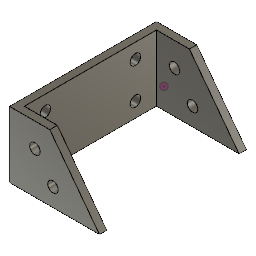
updated_housing_clamp_for_motor v3 (Autodesk Fusion 360 design; units mm, degrees)
Autodesk Fusion 360 part; units mm, degrees
note: some values were not read from the file. Chosen so that the rebuilt part matches the saved one: which face or edge a step refers to.
sketch "Sketch1" plane through (0, 0, 0) normal (0, 0, 1) x (1, 0, 0)
  line L0 (0, 0) -> (2, 0)
  line L1 (0, -2) -> (0, 0)
  line L2 (2, -2) -> (42, -2)
  line L3 (42, -2) -> (42, -24)
  line L4 (42, -24) -> (2, -24)
  line L5 (2, -24) -> (2, -2)
  line L6 (44, -24) -> (44, -26)
  line L7 (44, -26) -> (42, -26)
  line L8 (0, 0) -> (44, 0)
  line L9 (44, 0) -> (44, -26)
  line L10 (44, -26) -> (0, -26)
  line L11 (0, -26) -> (0, 0)
  dimension "d1" = 2
  dimension "d2" = 2
  dimension "d3" = 22
  dimension "d4" = 40
  dimension "d5" = 2
  dimension "d6" = 2
  measures "d1" distance of L0.start
  measures "d2" distance of L0.start
sketch "Sketch2" plane through (0, 0, 0) normal (0, 0, 1) x (1, 0, 0)
  line L0 (0, -26) -> (44, -26)
  line L1 (44, -26) -> (44, 0)
  line L2 (44, 0) -> (0, 0)
  line L3 (0, 0) -> (0, -26)
sketch "Sketch3" plane through (0, 0, -2) normal (0, 0, -1) x (1, 0, 0)
  line L0 (0, 26) -> (0, 0)
  line L1 (0, 0) -> (44, 0)
  line L2 (44, 0) -> (44, 26)
  line L3 (44, 26) -> (0, 26)
  line L4 (0, 0) -> (7, 0)
  line L5 (7, 0) -> (7, 7)
  line L6 (7, 7) -> (0, 7)
  line L7 (0, 7) -> (0, 0)
  dimension "d11" = 7
  dimension "d12" = 7
  measures "d11" distance of L0.end
  measures "d12" distance of L0.end
sketch "Sketch4" plane through (0, 0, -2) normal (0, 0, -1) x (1, 0, 0)
  circle A0 centre (7, 7) radius 1.5
  line L0 (0, 26) -> (0, 0)
  line L1 (0, 0) -> (44, 0)
  line L2 (44, 0) -> (44, 26)
  line L3 (44, 26) -> (0, 26)
  line L4 (44, 0) -> (37, 0)
  line L5 (37, 0) -> (37, 7)
  line L6 (37, 7) -> (44, 7)
  line L7 (44, 7) -> (44, 0)
  dimension "d16" = 7
  dimension "d17" = 7
  measures "d16" distance of L0.end
sketch "Sketch5" plane through (0, 0, -2) normal (0, 0, -1) x (1, 0, 0)
  circle A0 centre (37, 7) radius 1.5
  circle A1 centre (7, 7) radius 1.5
  line L0 (0, 26) -> (0, 0)
  line L1 (0, 0) -> (44, 0)
  line L2 (44, 0) -> (44, 26)
  line L3 (44, 26) -> (0, 26)
  line L4 (0, 26) -> (7, 26)
  line L5 (7, 26) -> (7, 19)
  line L6 (7, 19) -> (0, 19)
  line L7 (0, 19) -> (0, 26)
  dimension "d21" = 7
  dimension "d22" = 7
  measures "d21" distance of L0.end
  measures "d22" distance of L0.end
sketch "Sketch6" plane through (0, 0, -2) normal (0, 0, -1) x (1, 0, 0)
  circle A0 centre (7, 19) radius 1.5
  circle A1 centre (37, 7) radius 1.5
  circle A2 centre (7, 7) radius 1.5
  line L0 (0, 26) -> (0, 0)
  line L1 (0, 0) -> (44, 0)
  line L2 (44, 0) -> (44, 26)
  line L3 (44, 26) -> (0, 26)
  line L4 (44, 26) -> (37, 26)
  line L5 (37, 26) -> (37, 19)
  line L6 (37, 19) -> (44, 19)
  line L7 (44, 19) -> (44, 26)
  dimension "d26" = 7
  dimension "d27" = 7
  measures "d27" distance of L0.end
ref_plane "WorkPlane1" through (22, -26, 105) normal (0, 0.838671, 0.544639) x (1, 0, 0)
sketch "Sketch7" plane through (22, -26, 105) normal (0, 0.838671, 0.544639) x (1, 0, 0)
sketch "Sketch8" plane through (44, 0, 0) normal (1, 0, 0) x (0, 1, 0)
sketch "Sketch9" plane through (0, 0, -2) normal (0, 0, -1) x (1, 0, 0)
sketch "Sketch10" plane through (0, 0, 0) normal (0, 0, 1) x (1, 0, 0)
  line L0 (-69, 0) -> (-25, 0)
  line L1 (-25, 0) -> (-25, -26)
  line L2 (-25, -26) -> (-69, -26)
  line L3 (-69, -26) -> (-69, 0)
  dimension "d40" = 44
  dimension "d41" = 26
extrude "Extrude3" add sketch "Sketch10" against normal blind 2
sketch "Sketch11" plane through (0, 0, 0) normal (0, 0, 1) x (-1, 0, 0)
  line L0 (69, 26) -> (25, 26)
  line L1 (25, 26) -> (25, 0)
  line L2 (25, 0) -> (69, 0)
  line L3 (69, 0) -> (69, 26)
  line L4 (69, 26) -> (62, 26)
  line L5 (62, 26) -> (62, 19)
  line L6 (62, 19) -> (69, 19)
  line L7 (69, 19) -> (69, 26)
  dimension "d44" = 7
  dimension "d45" = 7
  measures "d45" distance of origin
hole "Hole5" at (-62, -19, 0) direction (0, 0, -1) diameter 3 depth 19 tip angle 118
sketch "Sketch12" plane through (0, 0, 0) normal (0, 0, 1) x (-1, 0, 0)
  circle A0 centre (62, 19) radius 1.5
  line L0 (69, 26) -> (25, 26)
  line L1 (25, 26) -> (25, 0)
  line L2 (25, 0) -> (69, 0)
  line L3 (69, 0) -> (69, 26)
  line L4 (69, 0) -> (62, 0)
  line L5 (62, 0) -> (62, 7)
  line L6 (62, 7) -> (69, 7)
  line L7 (69, 7) -> (69, 0)
  dimension "d49" = 7
  dimension "d50" = 7
  measures "d50" distance of origin
hole "Hole6" at (-62, -7, 0) direction (0, 0, -1) diameter 3 depth 19 tip angle 118
sketch "Sketch13" plane through (0, 0, 0) normal (0, 0, 1) x (-1, 0, 0)
  circle A0 centre (62, 7) radius 1.5
  circle A1 centre (62, 19) radius 1.5
  line L0 (69, 26) -> (25, 26)
  line L1 (25, 26) -> (25, 0)
  line L2 (25, 0) -> (69, 0)
  line L3 (69, 0) -> (69, 26)
  line L4 (25, 26) -> (32, 26)
  line L5 (32, 26) -> (32, 19)
  line L6 (32, 19) -> (25, 19)
  line L7 (25, 19) -> (25, 26)
  dimension "d54" = 7
  dimension "d55" = 7
  measures "d55" distance of origin
hole "Hole7" at (-32, -19, 0) direction (0, 0, -1) diameter 3 depth 19 tip angle 118
sketch "Sketch14" plane through (0, 0, 0) normal (0, 0, 1) x (-1, 0, 0)
  circle A0 centre (32, 19) radius 1.5
  circle A1 centre (62, 7) radius 1.5
  circle A2 centre (62, 19) radius 1.5
  line L0 (69, 26) -> (25, 26)
  line L1 (25, 26) -> (25, 0)
  line L2 (25, 0) -> (69, 0)
  line L3 (69, 0) -> (69, 26)
  line L4 (25, 0) -> (32, 0)
  line L5 (32, 0) -> (32, 7)
  line L6 (32, 7) -> (25, 7)
  line L7 (25, 7) -> (25, 0)
  dimension "d59" = 7
  dimension "d60" = 7
  measures "d60" distance of origin
hole "Hole8" at (-32, -7, 0) direction (0, 0, -1) diameter 3 depth 19 tip angle 118
extrude "Extrude4" add 1 faces at (-69, -17.3333, -0.6667) along direction (-1, 0, 0) blind 0.5
extrude "Extrude5" add 1 faces at (-25, -8.6667, -0.6667) along direction (1, 0, 0) blind 0.5
sketch "Sketch15" plane through (0, 0, -2) normal (0, 0, -1) x (1, 0, 0)
  circle A0 centre (-32, 7) radius 1.5
  circle A1 centre (-32, 19) radius 1.5
  circle A2 centre (-62, 7) radius 1.5
  circle A3 centre (-62, 19) radius 1.5
  line L0 (-24.5, 26) -> (-69.5, 26)
  line L1 (-69.5, 26) -> (-69.5, 0)
  line L2 (-69.5, 0) -> (-24.5, 0)
  line L3 (-24.5, 0) -> (-24.5, 26)
  line L4 (-69.5, 26) -> (-71.5, 26)
  line L5 (-71.5, 26) -> (-71.5, 0)
  line L6 (-71.5, 0) -> (-69.5, 0)
  line L7 (-69.5, 0) -> (-69.5, 26)
  line L8 (-24.5, 26) -> (-22.5, 26)
  line L9 (-22.5, 26) -> (-22.5, 0)
  line L10 (-22.5, 0) -> (-24.5, 0)
  line L11 (-24.5, 0) -> (-24.5, 26)
  dimension "d68" = 2
  dimension "d69" = 2
extrude "Extrude6" add sketch "Sketch15" against normal blind 20 contours L3 L8 L9 L10 L11 | L1 L4 L5 L6 L7
sketch "Sketch16" plane through (0, -0.0046, 103.0012) normal (0, -0.000045, 1) x (1, 0, 0)
  line L0 (44, -25.9961) -> (44, -13.9759)
  line L1 (44, -13.9759) -> (42, -13.9759)
  line L2 (42, -13.9759) -> (42, -23.9961)
  line L3 (42, -23.9961) -> (2, -23.9961)
  line L4 (2, -23.9961) -> (2, -13.9759)
  line L5 (2, -13.9759) -> (0, -13.9759)
  line L6 (0, -13.9759) -> (0, -25.9961)
  line L7 (0, -25.9961) -> (44, -25.9961)
  line L8 (44, -25.9961) -> (44, -0.0001)
  line L9 (44, -0.0001) -> (0, -0.0001)
  line L10 (0, -0.0001) -> (0, -25.9961)
  line L11 (2, -23.9961) -> (42, -23.9961)
  line L12 (42, -23.9961) -> (42, -2)
  line L13 (42, -2) -> (2, -2)
  line L14 (2, -2) -> (2, -23.9961)
  line L15 (0, -25.9961) -> (44, -25.9961)
extrude "Extrude9" cut 1 faces at (-42.4654, -14.8173, -2) along direction (0, 0.000045, -1) blind 39
delete_face "DeleteFace2" [no effect]
delete_face "DeleteFace3" [no effect]
sketch "Sketch17" plane through (44, 0, 0) normal (1, 0, 0) x (0, 1, 0)
sketch "Sketch18" plane through (44, 0, 0) normal (1, 0, 0) x (0, 1, 0)
  line L0 (-0.0003, 70.5005) -> (-26.0018, 105.0024)
  line L1 (-26.0018, 105.0024) -> (-1.7646, 105.0024) construction
  line L2 (-2, 73.1539) -> (-24, 56.5757)
  line L3 (-2, 73.1539) -> (25.547, 73.1539) construction
  line L4 (-26.0018, 105.0024) -> (-34.7623, 98.401)
  line L5 (-26.0018, 105.0024) -> (-4.2688, 105.0024) construction
  line L6 (-26.0018, 105.0024) -> (-2, 73.1539)
  line L7 (-34.7623, 98.401) -> (-28.1604, 89.6399)
  line L8 (-26.0018, 105.0024) -> (-26.001, 95.0024)
  line L9 (-26, 64) -> (0, 64.0012)
  line L10 (0, 64.0012) -> (-0.0003, 70.5005)
  line L11 (-26.0018, 105.0024) -> (-26, 64)
  dimension "d86" = 143
  dimension "d87" = 143
  dimension "d107" = 10.97
  dimension "d108" = 10
  measures "d86" angle of L2 L3
  measures "d87" angle of L4 L5
extrude "Extrude11" cut 1 faces at (-70.8333, -17.3333, 18) along direction (0, 0, -1) blind 18
extrude "Extrude12" cut 1 faces at (-23.1667, -8.6667, 18) along direction (0, 0, -1) blind 18
sketch "Sketch19" plane through (-71.5, 0, 0) normal (-1, 0, 0) x (0, -1, 0)
extrude "Extrude13" cut 1 faces at (-38.8333, 0, -1.3333) along direction (0, -1, 0) blind 2
extrude "Extrude14" cut 1 faces at (-38.8333, -26, -0.6667) along direction (0, 1, 0) blind 2
sketch "Sketch20" plane through (-71.5, 0, 0) normal (-1, 0, 0) x (0, -1, 0)
  line L0 (24, -2) -> (24, 0)
  line L1 (24, 0) -> (2, 0)
  line L2 (2, 0) -> (2, -2)
  line L3 (2, -2) -> (24, -2)
  line L4 (2, 0) -> (2, 27.55)
  line L5 (24, 0) -> (24, 10.97)
  line L6 (2, 27.55) -> (24, 10.97)
  dimension "d98" = 27.55
  dimension "d99" = 10.97
  measures "d99" distance of origin
extrude "Extrude15" add sketch "Sketch20" against normal blind 2 contours L1 L4 L5 L6
sketch "Sketch21" plane through (-22.5, 0, 0) normal (1, 0, 0) x (0, 1, 0)
  line L0 (-24, 0) -> (-24, -2)
  line L1 (-24, -2) -> (-2, -2)
  line L2 (-2, -2) -> (-2, 0)
  line L3 (-2, 0) -> (-24, 0)
  line L4 (-24, 0) -> (-24, 10.97)
  line L5 (-2, 0) -> (-2, 27.55)
  line L6 (-2, 27.55) -> (-24, 10.97)
  dimension "d102" = 10.97
  dimension "d104" = 27.55
  measures "d102" distance of origin
extrude "Extrude16" add sketch "Sketch21" against normal blind 2 contours L3 L4 L5 L6
sketch "Sketch22" plane through (-71.5, 0, 0) normal (-1, 0, 0) x (0, -1, 0)
  line L0 (24, -2) -> (24, 10.97)
  line L1 (24, 10.97) -> (2, 27.55)
  line L2 (2, 27.55) -> (2, -2)
  line L3 (2, -2) -> (24, -2)
  line L4 (24, 0) -> (16.0136, 6.0182)
  line L5 (24, 0) -> (14, 0) construction
  dimension "d112" = 37
  dimension "d113" = 10
  measures "d112" angle of L4 L5
  measures "d113" distance of origin
sketch "Sketch23" plane through (-22.5, 0, 0) normal (1, 0, 0) x (0, 1, 0)
  line L0 (-24, 10.97) -> (-24, -2)
  line L1 (-24, -2) -> (-2, -2)
  line L2 (-2, -2) -> (-2, 27.55)
  line L3 (-2, 27.55) -> (-24, 10.97)
  line L4 (-24, 0) -> (-16.0136, 6.0182)
  line L5 (-24, 0) -> (-14, 0) construction
  dimension "d117" = 37
  measures "d117" angle of L4 L5
sketch "Sketch24" plane through (0, 0, 0) normal (-1, 0, 0) x (0, -1, 0)
  line L0 (26.0018, 105.0024) -> (0.0003, 70.5005)
  line L1 (26.0018, 105.0024) -> (26.001, 95.0024)
  line L2 (0, 64.0012) -> (26, 64)
  line L3 (26, 64) -> (26.0018, 105.0024)
  line L4 (0.0003, 70.5005) -> (0, 64.0012)
  dimension "d121" = 10
sketch "Sketch25" plane through (44, 0, 0) normal (1, 0, 0) x (0, 1, 0)
  line L0 (-0.0003, 70.5005) -> (-26.0018, 105.0024)
  line L1 (-24, 0) -> (-24, 90.7202)
  line L2 (-2, 73.1539) -> (-24, 56.5757)
  line L3 (-2, 73.1539) -> (25.547, 73.1539) construction
  line L4 (-15.2381, 80.7209) -> (-15.2381, 70.7209)
  arc A0 (-26.0013, 93.5024) -> (-26.0015, 96.5024) centre (-26.001, 95.0024) ccw
  line L5 (-26.0013, 93.5024) -> (-26, 64)
  line L6 (-26, 64) -> (0, 64.0012)
  line L7 (0, 64.0012) -> (-0.0003, 70.5005)
  line L8 (-26.0018, 105.0024) -> (-26.0015, 96.5024)
  dimension "d125" = 143
  dimension "d126" = 10
  measures "d125" angle of L2 L3
sketch "Sketch26" plane through (0, 0, 0) normal (-1, 0, 0) x (0, -1, 0)
  line L0 (26.0018, 105.0024) -> (0.0003, 70.5005)
  line L1 (15.2381, 80.7209) -> (15.2381, 70.7209)
  arc A0 (26.0015, 96.5024) -> (26.0013, 93.5024) centre (26.001, 95.0024) ccw
  line L2 (26.0015, 96.5024) -> (26.0018, 105.0024)
  line L3 (0.0003, 70.5005) -> (0, 64.0012)
  line L4 (0, 64.0012) -> (26, 64)
  line L5 (26, 64) -> (26.0013, 93.5024)
  dimension "d130" = 10
sketch "Sketch27" plane through (-71.5, 0, 0) normal (-1, 0, 0) x (0, -1, 0)
  line L0 (24, -2) -> (24, 10.97)
  line L1 (24, 10.97) -> (2, 27.55)
  line L2 (2, 27.55) -> (2, -2)
  line L3 (2, -2) -> (24, -2)
  line L4 (24, 0) -> (16.0136, 6.0182)
  line L5 (16.0136, 6.0182) -> (8.0273, 12.0363)
  dimension "d134" = 10
sketch "Sketch28" plane through (-22.5, 0, 0) normal (1, 0, 0) x (0, 1, 0)
  line L0 (-24, 10.97) -> (-24, -2)
  line L1 (-24, -2) -> (-2, -2)
  line L2 (-2, -2) -> (-2, 27.55)
  line L3 (-2, 27.55) -> (-24, 10.97)
  line L4 (-24, 0) -> (-16.0136, 6.0182)
  line L5 (-16.0136, 6.0182) -> (-8.0273, 12.0363)
  dimension "d138" = 10
move_body "Move1" bodies 1 to x (1, 0, 0) y (0, 0, -1) z (0, 1, 0) at (0, 0, -4)
sketch "Sketch29" plane through (-22.5, 0, 0) normal (1, 0, 0) x (0, 1, 0)
  line L0 (10.97, 20) -> (-2, 20)
  line L1 (-2, 20) -> (-2, -2)
  line L2 (-2, -2) -> (27.55, -2)
  line L3 (27.55, -2) -> (10.97, 20)
  line L4 (0, 20) -> (6.0182, 12.0136)
  line L5 (6.0182, 12.0136) -> (12.0363, 4.0273)
  dimension "d144" = 10
hole "Hole17" at (-22.5, 12.0363, 4.0273) direction (-1, 0, 0) diameter 3.5 depth 6 tip angle 118
sketch "Sketch30" plane through (-22.5, 0, 0) normal (1, 0, 0) x (0, 1, 0)
  circle A0 centre (12.0363, 4.0273) radius 1.75
  line L0 (10.97, 20) -> (-2, 20)
  line L1 (-2, 20) -> (-2, -2)
  line L2 (-2, -2) -> (27.55, -2)
  line L3 (27.55, -2) -> (10.97, 20)
  line L4 (0, 20) -> (6.0182, 12.0136)
  line L5 (0, 20) -> (10, 20) construction
  dimension "d148" = 53
  dimension "d149" = 10
  measures "d148" angle of L4 L5
hole "Hole18" at (-22.5, 6.0182, 12.0136) direction (-1, 0, 0) diameter 3.5 depth 3.5 tip angle 118
sketch "Sketch31" plane through (-71.5, 0, 0) normal (-1, 0, 0) x (0, -1, 0)
  line L0 (2, 20) -> (-10.97, 20)
  line L1 (-10.97, 20) -> (-27.55, -2)
  line L2 (-27.55, -2) -> (2, -2)
  line L3 (2, -2) -> (2, 20)
  line L4 (0, 20) -> (-6.0182, 12.0136)
  line L5 (-6.0182, 12.0136) -> (-12.0363, 4.0273)
  dimension "d153" = 10
hole "Hole19" at (-71.5, 12.0363, 4.0273) direction (1, 0, 0) diameter 3.5 depth 3.5 tip angle 118
sketch "Sketch32" plane through (-71.5, 0, 0) normal (-1, 0, 0) x (0, -1, 0)
  circle A0 centre (-12.0363, 4.0273) radius 1.75
  line L0 (2, 20) -> (-10.97, 20)
  line L1 (-10.97, 20) -> (-27.55, -2)
  line L2 (-27.55, -2) -> (2, -2)
  line L3 (2, -2) -> (2, 20)
  line L4 (0, 20) -> (-6.0182, 12.0136)
  line L5 (0, 20) -> (10, 20) construction
  dimension "d157" = 127
  dimension "d158" = 10
  measures "d157" angle of L4 L5
hole "Hole20" at (-71.5, 6.0182, 12.0136) direction (1, 0, 0) diameter 3.5 depth 3.5 tip angle 118
sketch "Sketch33" plane through (0, -2, 0) normal (0, -1, 0) x (1, 0, 0)
  line L0 (-22.5, 20) -> (-71.5, 20)
  line L1 (-71.5, 20) -> (-71.5, -2)
  line L2 (-71.5, -2) -> (-22.5, -2)
  line L3 (-22.5, -2) -> (-22.5, 20)
  circle A0 centre (-62, 15) radius 1.5
  circle A1 centre (-62, 3) radius 1.5
  circle A2 centre (-32, 15) radius 1.5
  circle A3 centre (-32, 3) radius 1.5
  line L4 (-62, 3) -> (-62, 15)
hole "Hole21" at (-62, -2, 15) direction (0, 1, 0) diameter 3.5 depth 3.5 tip angle 118
sketch "Sketch34" plane through (0, -2, 0) normal (0, -1, 0) x (1, 0, 0)
  circle A0 centre (-62, 15) radius 1.75
  line L0 (-22.5, 20) -> (-71.5, 20)
  line L1 (-71.5, 20) -> (-71.5, -2)
  line L2 (-71.5, -2) -> (-22.5, -2)
  line L3 (-22.5, -2) -> (-22.5, 20)
  circle A1 centre (-62, 3) radius 1.5
  circle A2 centre (-32, 15) radius 1.5
  circle A3 centre (-32, 3) radius 1.5
  line L4 (-62, 15) -> (-62, 3)
hole "Hole22" at (-62, -2, 3) direction (0, 1, 0) diameter 3.5 depth 3.5 tip angle 118
sketch "Sketch35" plane through (0, -2, 0) normal (0, -1, 0) x (1, 0, 0)
  circle A0 centre (-62, 3) radius 1.75
  circle A1 centre (-62, 15) radius 1.75
  line L0 (-22.5, 20) -> (-71.5, 20)
  line L1 (-71.5, 20) -> (-71.5, -2)
  line L2 (-71.5, -2) -> (-22.5, -2)
  line L3 (-22.5, -2) -> (-22.5, 20)
  circle A2 centre (-32, 15) radius 1.5
  circle A3 centre (-32, 3) radius 1.5
  line L4 (-32, 15) -> (-32, 3)
hole "Hole23" at (-32, -2, 3) direction (0, 1, 0) diameter 3.5 depth 3.5 tip angle 118
sketch "Sketch36" plane through (0, -2, 0) normal (0, -1, 0) x (1, 0, 0)
  circle A0 centre (-32, 3) radius 1.75
  circle A1 centre (-62, 3) radius 1.75
  circle A2 centre (-62, 15) radius 1.75
  line L0 (-22.5, 20) -> (-71.5, 20)
  line L1 (-71.5, 20) -> (-71.5, -2)
  line L2 (-71.5, -2) -> (-22.5, -2)
  line L3 (-22.5, -2) -> (-22.5, 20)
  circle A3 centre (-32, 15) radius 1.5
  line L4 (-32, 3) -> (-32, 15)
hole "Hole24" at (-32, -2, 15) direction (0, 1, 0) diameter 3.5 depth 3.5 tip angle 118
extrude "Extrude17" add 1 faces at (-51.457, -2, 7.2131) along direction (0, -1, 0) blind 0.5
extrude "Extrude18" add 1 faces at (-69.5, 17.3082, 7.7061) along direction (1, 0, 0) blind 0.5
extrude "Extrude19" add 1 faces at (-24.5, 17.3082, 7.7061) along direction (-1, 0, 0) blind 0.5
move_body "Move2" bodies 1 to x (0, -1, 0) y (1, 0, 0) z (0, 0, 1) at (-69, -74, 0)
